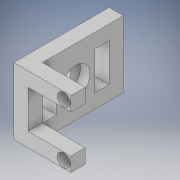
# Autodesk Inventor part: TensionerPlate
Saved by Autodesk Inventor 2017 (Build 210142000, 142)
## iProperties
Created: 2017-07-29
Part Number: TensionerPlate
Material: Generic
Document SubType Name: Modeling
Designer: User
Density: 1 g/cm^3
Appearance: Default
Author: User
Autodesk Inventor part; units mm, degrees
ref_plane "YZ Plane" through (0, 0, 0) normal (1, 0, 0) x (0, 1, 0)
ref_plane "XZ Plane" through (0, 0, 0) normal (0, 1, 0) x (-1, 0, 0)
ref_plane "XY Plane" through (0, 0, 0) normal (0, 0, 1) x (1, 0, 0)
sketch "Sketch1" plane through (0, 0, 0) normal (1, 0, 0) x (0, 1, 0)
  line L0 (22.225, 0) -> (22.225, -31.75)
  line L1 (22.225, -31.75) -> (0, -31.75)
  line L2 (0, -31.75) -> (0, 0)
  line L3 (17.4625, -4.7625) -> (4.7625, -4.7625)
  line L4 (6.35, -31.75) -> (25.4, -31.75)
  line L5 (0, 0) -> (4.7625, 0)
  line L6 (17.4625, 0) -> (22.225, 0)
  line L7 (4.7625, -22.225) -> (17.4625, -22.225)
  line L8 (17.4625, -22.225) -> (17.4625, -26.9875)
  line L9 (17.4625, -26.9875) -> (4.7625, -26.9875)
  line L10 (4.7625, -26.9875) -> (4.7625, -22.225)
  line L11 (22.225, 0) -> (0, 0)
  line L12 (17.4625, -4.7625) -> (4.7625, -4.7625)
  line L13 (4.7625, -4.7625) -> (4.7625, -9.525)
  line L14 (4.7625, -9.525) -> (17.4625, -9.525)
  line L15 (17.4625, -9.525) -> (17.4625, -4.7625)
  dimension "d8" = 12.7
  dimension "d9" = 4.7625
  dimension "d10" = 4.7625
  dimension "d11" = 4.7625
  dimension "d28" = 4.7625
  dimension "d29" = 4.7625
  dimension "d37" = 31.75
  dimension "d38" = 31.75
  dimension "d43" = 4.7625
  dimension "d48" = 12.7
  dimension "d49" = 4.7625
  constraints: 32 end point, 7 parallel, 5 horizontal, 4 perpendicular, 1 point on line
  measures "d8" distance of L8.end L9.end
  measures "d9" distance of L7.end L8.end
  measures "d10" distance between parallel lines of L1 L9
  measures "d11" distance between parallel lines of L2 L10
  measures "d28" distance between parallel lines of L8 L0
  measures "d29" distance of L6.start L3.start
  measures "d37" distance of L0.start L0.end
  measures "d38" distance of L1.end L2.end
  measures "d43" distance of L14.end L3.start
  measures "d48" distance of L13.end L14.end
  measures "d49" distance between parallel lines of L2 L13
extrude "Extrusion1" add sketch "Sketch1" along normal blind 4.7625 contours L0 L1 L2 L5 L11 L6 | L15 L14 L13 L3
sketch "Sketch2" plane through (4.7625, 0, 0) normal (1, 0, 0) x (0, 0, -1)
  line L0 (22.225, 17.4625) -> (26.9875, 17.4625) projected
  line L1 (26.9875, 17.4625) -> (26.9875, 4.7625) projected
  line L2 (26.9875, 4.7625) -> (22.225, 4.7625) projected
  line L3 (22.225, 4.7625) -> (22.225, 17.4625) projected
  line L4 (0, 0) -> (31.75, 0) projected
  line L5 (31.75, 0) -> (31.75, 22.225) projected
  line L6 (31.75, 22.225) -> (0, 22.225) projected
  circle A0 centre (15.875, 11.1125) radius 4.7625
  line L7 (0, 22.225) -> (0, 0) projected
  dimension "d14" = 9.525
  dimension "d15" = 11.1125
  dimension "d39" = 22.225
  dimension "d52" = 31.75
  dimension "d53" = 15.875
  constraints: 1 centre point
  measures "d14" diameter of A0
  measures "d15" distance from line of L6 A0.centre
  measures "d39" distance of L4.end L5.end
  measures "d52" distance of L5.end L6.end
  measures "d53" distance from line of L7 A0.centre
extrude "Extrusion2" cut sketch "Sketch2" against normal blind 3.175 contours A0
sketch "Sketch3" plane through (0, 0, 0) normal (0, 0, 1) x (1, 0, 0)
  line L0 (0, 22.225) -> (0, 4.9893)
  line L1 (0, 22.225) -> (6.35, 22.225)
  line L2 (0, 4.7625) -> (0, 0)
  line L3 (0, 0) -> (6.35, 0)
  line L4 (0, 4.7625) -> (6.35, 4.7625)
  line L5 (0, 22.225) -> (19.05, 22.225)
  line L6 (19.05, 22.225) -> (19.05, 17.4625)
  line L7 (19.05, 17.4625) -> (0, 17.4625)
  line L8 (0, 17.4625) -> (0, 22.225)
  circle A0 centre (16.6688, 19.8437) radius 2.159
  circle A1 centre (16.6688, 2.3813) radius 2.159
  line L9 (0, 0) -> (19.05, 0)
  line L10 (19.05, 0) -> (19.05, 4.7625)
  line L11 (19.05, 4.7625) -> (0, 4.7625)
  line L12 (0, 4.7625) -> (0, 0)
  line L13 (0, 22.225) -> (0, 0) projected
  line L14 (0, 0) -> (4.7625, 0) projected
  line L15 (4.7625, 22.225) -> (4.7625, 0) projected
  line L16 (0, 22.225) -> (4.7625, 22.225) projected
  point P0 (0, -17.4625)
  dimension "d21" = 19.05
  dimension "d22" = 4.318
  dimension "d23" = 2.3813
  dimension "d24" = 4.318
  dimension "d33" = 19.05
  dimension "d34" = 2.3813
  dimension "d35" = 2.3813
  dimension "d44" = 0
  dimension "d45" = 4.7625
  dimension "d46" = 2.3813
  dimension "d47" = 0
  constraints: 26 end point, 4 parallel, 2 centre point, 2 horizontal, 2 perpendicular
  measures "d21" distance of L6.end L7.end
  measures "d22" diameter of A0
  measures "d23" distance from line of L6 A0.centre
  measures "d24" diameter of A1
  measures "d33" distance of L2.start L10.end
  measures "d34" distance from line of L11 A1.centre
  measures "d35" distance from line of L10 A1.centre
  measures "d44" distance between parallel lines of L16 L5
  measures "d45" distance of L5.end L6.end
  measures "d46" distance from line of L7 A0.centre
  measures "d47" distance between parallel lines of L14 L9
extrude "Extrusion3" add sketch "Sketch3" against normal blind 4.7625 contours L1 L15 L7 L0 | L1 L5 L6 L7 L15 | L4 L15 L3 L2 | L4 L11 L10 L9 L3 L15
sketch "Sketch4" plane through (4.7625, 0, 0) normal (1, 0, 0) x (0, 0, -1)
  line L0 (4.7625, 0) -> (31.75, 0) projected
  line L1 (31.75, 0) -> (31.75, 22.225) projected
  line L2 (31.75, 22.225) -> (4.7625, 22.225) projected
  line L3 (22.225, 17.4625) -> (26.9875, 17.4625) projected
  line L4 (26.9875, 17.4625) -> (26.9875, 4.7625) projected
  line L5 (26.9875, 4.7625) -> (22.225, 4.7625) projected
  line L6 (22.225, 4.7625) -> (22.225, 17.4625) projected
  circle A0 centre (15.875, 11.1125) radius 4.7625 projected
  circle A1 centre (15.875, 11.1125) radius 1.5875
  line L7 (0, 17.4625) -> (0, 4.7625) projected
  line L8 (4.7625, 4.7625) -> (4.7625, 0) projected
  line L9 (4.7625, 22.225) -> (4.7625, 17.4625) projected
  line L10 (4.7625, 17.4625) -> (0, 17.4625) projected
  line L11 (0, 4.7625) -> (4.7625, 4.7625) projected
  point P0 (0, 0)
  dimension "d40" = 3.175
  constraints: 1 centre point, 1 coincident
  measures "d40" diameter of A1
extrude "Extrusion4" cut sketch "Sketch4" against normal blind 25.4 contours A1
extrude "Extrusion5" cut sketch "Sketch1" along normal blind 25.4 contours L15 L14 L13 L3
equation "\"d38\" = d37"
equation "\"d15\" = 0.5 * d39"
equation "\"d53\" = 0.5 * d52"
equation "\"d23\" = d46"
equation "\"d34\" = d46"
equation "\"d35\" = d23"
equation "\"d46\" = 0.5 * d45"
equation "\"d32\" = 0.5 * d31"
equation "\"d31\" = 6.274854"
body "Solid1"
